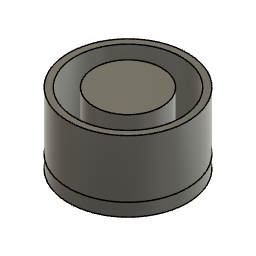
Rosita (Molde rueda siliciona) v1 (posible) (Autodesk Fusion 360 design; units mm, degrees)
Autodesk Fusion 360 part; units mm, degrees
note: some values were not read from the file. Chosen so that the rebuilt part matches the saved one: which bodies a step acts on.
sketch "Boceto1" plane through (0, 0, 0) normal (0, 1, 0) x (1, 0, 0)
  circle A0 centre (0, 0) radius 5.25
  circle A1 centre (0, 0) radius 8.25
  circle A2 centre (0, 0) radius 9.25
  dimension "d1" = 10.5
  dimension "d3" = 3
  dimension "d4" = 4
  constraint coincident A0.centre A1.centre
  measures "d1" diameter of A0
extrude "Extruir1" add sketch "Boceto1" along normal blind 2 contours A0 | A1 | A2 makes body 1
ref_plane "PlanoDeObra1" through (0, 2, 0) normal (0, 1, 0) x (1, 0, 0)
sketch "Boceto2" plane through (0, 2, 0) normal (0, 1, 0) x (1, 0, 0)
  circle A0 centre (0, 0) radius 8.9
  circle A1 centre (0, 0) radius 8.5
  dimension "d12" = 17.8
  dimension "d13" = 17
  constraint coincident A0.centre A1.centre
  constraint concentric A0 A1
  measures "d12" diameter of A0
  measures "d13" diameter of A1
extrude "Extruir5" add sketch "Boceto1" along normal blind 9 bodies 1
extrude "Extruir6" add sketch "Boceto1" against normal blind 2 contours A0 | A1 | A2 bodies 1
extrude "Extruir7" cut sketch "Boceto2" along normal blind 0.5 bodies 1
split "Dividir1" by plane through (0, 2, 0) normal (0, 1, 0) bodies 1 makes body 2 at (9.204, 4.3333, -0.921) makes body 3 at (5.2239, 4.3333, -0.5227)
combine "Combinar1" operation add target body 3 tool bodies 1
extrude "Extruir8" add sketch "Boceto2" along normal blind 0.5 bodies 3
extrude "Extruir9" add 1 faces at (-0.6975, 9, 2.4057) along direction (0, 1, 0) blind 2 on bodies 3 bodies 3
extrude "Extruir10" add 1 faces at (8.8515, 9, 0.8694) along direction (0, 1, 0) blind 2 on bodies 2 bodies 2
extrude "Extruir11" cut 1 faces at (-2.5312, -2, -3.8946) along direction (0, 1, 0) blind 2 on bodies 3 bodies 3
